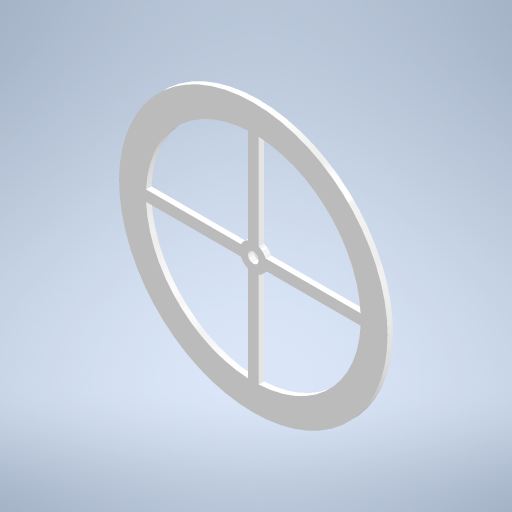
# Autodesk Inventor part: Seitenscheibe
Saved by Autodesk Inventor 2024.4 (Build 284460000, 460)
## iProperties
Created: 2026-01-10
Part Number: Seitenscheibe
Material: PVC, hart
Description: Seitenscheibe
Document SubType Name: Modeling
Designer: Philf
Mass: 373.258 g
Surface Area: 936.008 cm^2
Volume: 289.347 cm^3
Density: 1.29 g/cm^3
Appearance: Glatt - Weiß
Masse[kg]: 0,313 kg
nutlange: 210,000 mm
radius: 10,000 mm
Autodesk Inventor part; units mm, degrees
ref_plane "YZ Plane" through (0, 0, 0) normal (1, 0, 0) x (0, 1, 0)
ref_plane "XZ Plane" through (0, 0, 0) normal (0, 1, 0) x (-1, 0, 0)
ref_plane "XY Plane" through (0, 0, 0) normal (0, 0, 1) x (1, 0, 0)
sketch "Skizze1" plane through (0, 0, 0) normal (0, 1, 0) x (-1, 0, 0)
  circle A0 centre (0, 0) radius 10
  circle A1 centre (0, 0) radius 250
  circle A2 centre (0, 0) radius 200
  circle A3 centre (0, 0) radius 25
  line L0 (10, 0) -> (10, -249.7999)
  line L1 (-10, 0) -> (-10, -249.7999)
  line L2 (0, 10) -> (249.7999, 10)
  line L3 (0, -10) -> (249.7999, -10)
  line L4 (10, 0) -> (10, 249.7999)
  line L5 (-10, 0) -> (-10, 249.7999)
  line L6 (0, 10) -> (-199.7498, 10)
  line L7 (0, -10) -> (-199.7498, -10)
  point P0 (-10, -199.7498)
  point P1 (-22.9129, -10)
  point P2 (-10, -22.9129)
  point P3 (10, -199.7498)
  point P4 (10, -22.9129)
  point P5 (22.9129, -10)
  point P6 (199.7498, -10)
  point P7 (-10, 199.7498)
  point P8 (-10, 22.9129)
  point P9 (-22.9129, 10)
  point P10 (22.9129, 10)
  point P11 (10, 22.9129)
  point P12 (10, 199.7498)
  point P13 (199.7498, 10)
  dimension "d0" = 20
  dimension "d1" = 500
  dimension "d2" = 400
  dimension "d3" = 50
  constraints: 16 end point, 12 point on circle, 4 centre point, 4 coincident, 3 parallel, 3 perpendicular, 3 tangent, 2 vertical
  measures "d0" diameter of A0
  measures "d1" diameter of A1
  measures "d2" diameter of A2
  measures "d3" diameter of A3
extrude "Extrusion1" add sketch "Skizze1" along normal blind 10 contours L0 L3 A0 | L4 L2 A3 L3 L0 | A0 L2 L4 | L6 L5 A3 L4 L2 | A0 L5 L6 | L7 L1 A0 | L3 L0 A3 L1 L7 | L3 A3 L0 | L4 A3 L2 | L1 L7 A3 L6 L5 | L6 A3 L5 | L1 A3 L7 | L0 A2 L1 A3 | A3 L2 A2 L3 | A3 L5 A2 L4 | A3 L7 A2 L6 | L0 A1 L1 A2 | A2 L3 A1 L0 | A2 L2 A1 L3 | A2 L4 A1 L2 | A2 L5 A1 L4 | A2 L1 A1 L5
sketch "Skizze2" plane through (0, 10, 0) normal (0, 1, 0) x (1, 0, 0)
  line L0 (0, 22.9129) -> (0, 232.9129)
  circle A0 centre (0, 232.9129) radius 5
  circle A1 centre (0, 22.9129) radius 5
  line L1 (5, 232.9129) -> (5, 22.9129)
  line L2 (-5, 232.9129) -> (-5, 22.9129)
  line L3 (22.9129, 0) -> (232.9129, 0)
  circle A2 centre (232.9129, 0) radius 5
  circle A3 centre (22.9129, 0) radius 5
  line L4 (232.9129, -5) -> (22.9129, -5)
  line L5 (232.9129, 5) -> (22.9129, 5)
  line L6 (0, -22.9129) -> (0, -232.9129)
  circle A4 centre (0, -232.9129) radius 5
  circle A5 centre (0, -22.9129) radius 5
  line L7 (-5, -232.9129) -> (-5, -22.9129)
  line L8 (5, -232.9129) -> (5, -22.9129)
  line L9 (-22.9129, 0) -> (-232.9129, 0)
  circle A6 centre (-232.9129, 0) radius 5
  circle A7 centre (-22.9129, 0) radius 5
  line L10 (-232.9129, 5) -> (-22.9129, 5)
  line L11 (-232.9129, -5) -> (-22.9129, -5)
  point P0 (0, 0)
  point P1 (0, 0)
  point P2 (0, 0)
  point P3 (0, 0)
  dimension "nutlange" = 210
  dimension "radius" = 10
  dimension "d10" = 10
  dimension "d13" = 360
  constraints: 24 end point, 16 point on circle, 10 coincident, 8 centre point, 2 tangent, 1 vertical, 55 other
  measures "nutlange" distance of L0.start L0.end
  measures "radius" diameter of A0
  measures "d10" diameter of A1
extrude "Extrusion2" cut sketch "Skizze2" against normal blind 5
